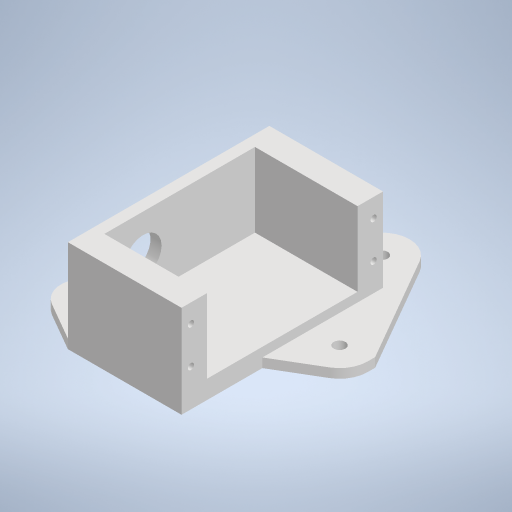
# Autodesk Inventor part: upper_arm_base
Saved by Autodesk Inventor 2024.1 (Build 281209000, 209)
## iProperties
Created: 2025-03-03
Part Number: upper_arm_base
Material: 一般
Document SubType Name: Modeling
Designer: hibik
Density: 1 g/cm^3
Appearance: 既定
Author: hibik
Autodesk Inventor part; units mm, degrees
ref_plane "XZ Plane" through (0, 0, 0) normal (0, 1, 0) x (-1, 0, 0)
ref_plane "XY Plane" through (0, 0, 0) normal (0, 0, 1) x (1, 0, 0)
ref_plane "作業平面1" through (7.8, 0, 0) normal (1, 0, 0) x (0, 1, 0)
sketch "スケッチ1" plane through (7.8, 0, 0) normal (1, 0, 0) x (0, 1, 0)
  line L0 (0, 27.3) -> (-20.1, 27.3)
  line L1 (-20.1, 27.3) -> (-20.1, 20.4)
  line L2 (-20.1, 20.4) -> (0, 20.4)
  line L3 (0, 20.4) -> (0, 27.3)
  line L4 (0, -20.4) -> (-20.1, -20.4)
  line L5 (-20.1, -20.4) -> (-20.1, -27.3)
  line L6 (-20.1, -27.3) -> (0, -27.3)
  line L7 (0, -27.3) -> (0, -20.4)
  line L8 (0, -38.22) -> (0, 38.22) projected
  line L9 (-24.12, 0) -> (4.02, 0) projected
  point P0 (0, 0)
  dimension "d1" = 40.8
  dimension "d3" = 20.1
  dimension "d13" = 6.9
  constraints: 16 end point, 4 parallel, 3 collinear, 2 horizontal, 2 perpendicular, 1 point on line, 1 other
  measures "d1" distance between parallel lines of L4 L2
  measures "d3" distance of L5.end L6.end
  measures "d13" distance of L2.end L0.start
extrude "押し出し1" add sketch "スケッチ1" against normal blind 27.8
sketch "スケッチ2" plane through (-20, 0, 0) normal (-1, 0, 0) x (0, 0, 1)
  line L0 (27.3, 0) -> (27.3, -20.1) projected
  line L1 (-27.3, -20.1) -> (-20.4, -20.1) projected
  line L2 (27.3, 0) -> (-27.3, 0)
  line L3 (-27.3, 0) -> (-27.3, -20.1)
  line L4 (-27.3, -20.1) -> (27.3, -20.1)
  line L5 (27.3, -20.1) -> (27.3, 0)
  point P0 (0, 0)
  constraints: 8 end point, 2 parallel, 1 horizontal, 1 perpendicular
extrude "押し出し2" add sketch "スケッチ2" along normal blind 3
sketch "スケッチ3" plane through (-23, 0, 0) normal (-1, 0, 0) x (0, 0, 1)
  circle A0 centre (9.9, -10.5) radius 5
  line L0 (27.3, 0) -> (-27.3, 0) projected
  line L1 (20.4, 0) -> (20.4, -20.1) projected
  point P0 (0, 0)
  dimension "d8" = 10
  dimension "d9" = 10.5
  dimension "d10" = 10.5
  constraints: 1 centre point
  measures "d8" diameter of A0
  measures "d9" distance from line of L0 A0.centre
  measures "d10" distance from line of L1 A0.centre
extrude "押し出し3" cut sketch "スケッチ3" against normal through all
sketch "スケッチ4" plane through (7.8, -20.1, -27.3) normal (0, -1, 0) x (1, 0, 0)
  line L0 (-7.8, -29.6912) -> (-7.8, 75.8281) construction
  line L1 (-36.96, 27.3) -> (6.16, 27.3) construction
  line L2 (-27.8, 42.2) -> (-27.8, 32.2) projected
  line L3 (-72.2412, 37.2) -> (44.4145, 37.2) construction
  line L4 (-59.5017, 67.05) -> (43.9017, 67.05)
  line L5 (43.9017, 67.05) -> (-7.8, -22.5)
  line L6 (-7.8, -22.5) -> (-59.5017, 67.05)
  line L7 (-59.5017, 67.05) -> (18.0509, 22.275) construction
  line L8 (43.9017, 67.05) -> (-33.6509, 22.275) construction
  line L9 (-30.8, 0) -> (-30.8, 54.6) projected
  line L10 (0, 0) -> (-30.8, 0) projected
  circle A0 centre (-7.8, -7.5) radius 7.5
  circle A1 centre (-7.8, -7.5) radius 1.6
  line L11 (0, 47.7) -> (-27.8, 47.7) projected
  line L12 (0, 6.9) -> (0, 0) projected
  line L13 (0, 54.6) -> (0, 47.7) projected
  line L14 (0, 54.6) -> (-30.8, 54.6) projected
  line L15 (15.2, 54.6) -> (15.2, 17.3372)
  line L16 (0, 54.6) -> (15.2, 54.6)
  circle A2 centre (-37.6196, 42.7882) radius 6.8196
  circle A3 centre (22.0196, 42.7882) radius 6.8196
  circle A4 centre (-37.6196, 42.7882) radius 1.6
  circle A5 centre (22.0196, 42.7882) radius 1.6
  line L17 (15.2, 54.6) -> (31.3353, 45.2843)
  line L18 (-30.8, 54.6) -> (-47.2104, 45.1254)
  circle A6 centre (7.6, 19.3736) radius 7.6
  line L19 (0, 47.7) -> (0, 54.6) projected
  circle A7 centre (7.6, 19.3736) radius 1.6
  line L20 (0, 54.6) -> (0, 32.6967)
  line L21 (11.4682, 25.9155) -> (0, 32.6967)
  point P0 (-7.8, 27.3)
  point P1 (-27.8, 37.2)
  point P2 (-7.8, 67.05)
  point P3 (-7.8, 37.2)
  point P4 (-7.8, 47.7)
  point P5 (-30.8, 17.3372)
  point P6 (-20.7904, 0)
  point P7 (-14.2952, -11.25)
  point P8 (-1.3048, -11.25)
  point P9 (0, 4.51)
  point P10 (-2.6038, 0)
  point P11 (-7.8, 0)
  point P12 (27.9255, 39.3784)
  point P13 (-43.5255, 39.3784)
  point P14 (15.2, 42.7882)
  point P15 (-30.8, 42.7882)
  point P16 (25.4294, 48.6941)
  point P17 (-41.0294, 48.6941)
  point P18 (15.2, 19.3736)
  dimension "d18" = 3.2
  dimension "d21" = 15
  constraints: 25 end point, 12 point on line, 8 tangent, 7 centre point, 4 coincident, 4 midpoint, 4 perpendicular, 3 equal radius, 3 horizontal, 2 equal length, 2 vertical, 6 other
  measures "d18" diameter of A1
  measures "d21" diameter of A0
extrude "押し出し4" add sketch "スケッチ4" along normal blind 5 contours A2 L9 L6 | A2 | L18 L9 A2 | L9 L14 L13 L20 L21 A6 L5 A0 L10 L6 | L6 L10 L9 | L5 A6 L15 | L10 A0 L6 | A6 | A0
sketch "スケッチ5" plane through (7.8, -20.1, -27.3) normal (0, 1, 0) x (1, 0, 0)
  line L0 (0, 0) -> (-20.7904, 0) projected
  line L1 (0, -6.9) -> (0, 0) projected
  line L2 (0, -6.9) -> (-27.8, -6.9) projected
  line L3 (-27.8, -6.9) -> (-27.8, -47.7) projected
  line L4 (0, -47.7) -> (-27.8, -47.7) projected
  line L5 (-1.3048, 11.25) -> (15.2, -17.3372) projected
  arc A0 (-1.3048, 11.25) -> (-14.2952, 11.25) centre (-7.8, 7.5) ccw projected
  line L6 (-20.7904, 0) -> (-14.2952, 11.25) projected
  circle A1 centre (7.6, -19.3736) radius 1.6 projected
  circle A2 centre (-7.8, 7.5) radius 1.6 projected
  line L7 (0, -47.7) -> (-27.8, -47.7)
  line L8 (-27.8, -47.7) -> (-27.8, -6.9)
  line L9 (-27.8, -6.9) -> (0, -6.9)
  line L10 (0, -6.9) -> (0, -47.7)
  line L11 (-30.8, -17.3372) -> (-30.8, -54.6) projected
  line L12 (-43.5255, -39.3784) -> (-30.8, -17.3372) projected
  arc A3 (-43.5255, -39.3784) -> (-41.0294, -48.6941) centre (-37.6196, -42.7882) ccw projected
  line L13 (-30.8, -54.6) -> (-41.0294, -48.6941) projected
  circle A4 centre (-37.6196, -42.7882) radius 1.6 projected
  line L14 (0, -32.6967) -> (0, -47.7) projected
  line L15 (11.4682, -25.9155) -> (0, -32.6967) projected
  arc A5 (11.4682, -25.9155) -> (15.2, -19.3736) centre (7.6, -19.3736) ccw projected
  line L16 (15.2, -17.3372) -> (15.2, -19.3736) projected
  point P0 (-7.8, -27.3)
  constraints: 8 end point, 2 parallel, 1 horizontal, 1 perpendicular
extrude "押し出し5" cut sketch "スケッチ5" against normal blind 2.5 contours L0 L6 A0 L5 L16 A5 L15 L10 L1 | L11 L13 A3 L12
sketch "スケッチ6" plane through (7.8, -22.6, -27.3) normal (0, 1, 0) x (1, 0, 0)
  point P0 (-7.8, -27.3)
sketch "スケッチ7" plane through (7.8, 0, 0) normal (1, 0, 0) x (0, 0, -1)
  arc A0 (-26.6208, -6.3) -> (-26.6208, -3.8) centre (-24.75, -5.05) ccw projected
  arc A1 (-26.6208, -16.3) -> (-26.6208, -13.8) centre (-24.75, -15.05) ccw projected
  arc A2 (26.6208, -3.8) -> (26.6208, -6.3) centre (24.75, -5.05) ccw projected
  arc A3 (26.6208, -13.8) -> (26.6208, -16.3) centre (24.75, -15.05) ccw projected
  circle A4 centre (-24.75, -5.05) radius 0.85
  circle A5 centre (-24.75, -15.05) radius 0.85
  circle A6 centre (24.75, -5.05) radius 0.85
  circle A7 centre (24.75, -15.05) radius 0.85
  point P0 (0, 0)
  dimension "d25" = 1.7
  constraints: 4 centre point, 3 coincident, 3 equal radius, 1 concentric
  measures "d25" diameter of A4
extrude "押し出し6" cut sketch "スケッチ7" against normal through all
